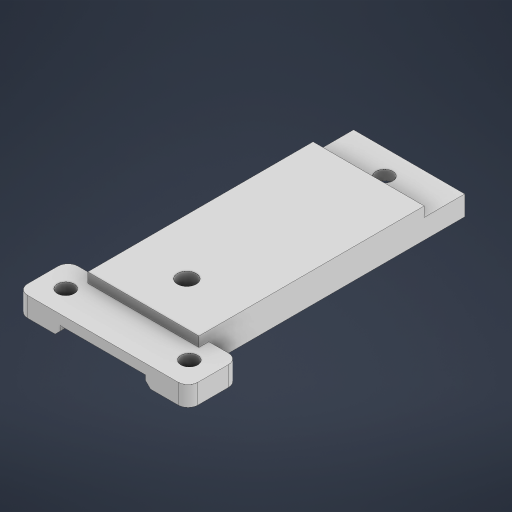
# Autodesk Inventor part: Zwischenplatte
Saved by Autodesk Inventor 2024.2 (Build 282272000, 272)
## iProperties
Created: 2024-01-03
Part Number: Zwischenplatte
Material: Generisch
Document SubType Name: Modeling
Designer: jacob
Density: 1 g/cm^3
Appearance: Vorgabe
Author: jacob
Autodesk Inventor part; units mm, degrees
ref_plane "YZ Plane" through (0, 0, 0) normal (1, 0, 0) x (0, 1, 0)
ref_plane "XZ Plane" through (0, 0, 0) normal (0, 1, 0) x (-1, 0, 0)
ref_plane "XY Plane" through (0, 0, 0) normal (0, 0, 1) x (1, 0, 0)
sketch "Skizze1" plane through (0, 0, 0) normal (0, 1, 0) x (-1, 0, 0)
  line L0 (17.75, 60) -> (-17.75, 60)
  line L1 (-17.75, 60) -> (-17.75, 0)
  line L2 (-17.75, 0) -> (17.75, 0)
  line L3 (17.75, 0) -> (17.75, 60)
  point P0 (0, 0)
  point P1 (0, 0)
  dimension "d0" = 60
  dimension "d1" = 35.5
  constraints: 8 end point, 2 coincident, 2 parallel, 1 horizontal, 1 midpoint, 1 perpendicular
  measures "d0" distance of L2.end L0.start
  measures "d1" distance of L0.start L0.end
extrude "Extrusion1" add sketch "Skizze1" along normal blind 2
sketch "Skizze3" plane through (0, 2, 0) normal (0, 1, 0) x (1, 0, 0)
  line L0 (-17.75, 0) -> (-17.75, -60) projected
  line L1 (17.75, -60) -> (17.75, 0) projected
  line L2 (-17.75, -51.8) -> (17.75, -51.8)
  line L3 (17.75, -51.8) -> (17.75, -6.2)
  line L4 (-17.75, -6.2) -> (-17.75, -51.8)
  line L5 (17.75, 0) -> (-17.75, 0) projected
  line L6 (-17.75, -6.2) -> (17.75, -6.2)
  point P0 (0, 0)
  point P1 (17.75, -51.8)
  point P2 (0, 0)
  dimension "d71" = 51.8
  dimension "d75" = 6.2
  constraints: 8 end point, 2 perpendicular, 2 point on line, 1 horizontal, 1 midpoint, 1 parallel
  measures "d71" distance between parallel lines of L5 L2
  measures "d75" distance from line of point (0, 0) L6
extrude "Extrusion3" add sketch "Skizze3" along normal blind 2 contours L6 L1 L2 L0
sketch "Skizze6" plane through (0, 0, 0) normal (0, -1, 0) x (1, 0, 0)
  line L0 (-17.75, 60) -> (17.75, 60) projected
  line L1 (11.25, 60) -> (-11.25, 60)
  line L2 (-11.25, 60) -> (-11.25, 0)
  line L3 (-11.25, 0) -> (11.25, 0)
  line L4 (11.25, 0) -> (11.25, 60)
  line L5 (8.65, 60) -> (-8.65, 60)
  line L6 (-8.65, 60) -> (-8.65, 0)
  line L7 (-8.65, 0) -> (8.65, 0)
  line L8 (8.65, 0) -> (8.65, 60)
  line L9 (0, -15.6) -> (0, 72.6) projected
  line L10 (17.75, 0) -> (-17.75, 0) projected
  point P0 (0, 0)
  point P1 (0, 60)
  point P2 (0, -1)
  point P3 (0, 60)
  point P4 (0, 0)
  point P5 (8.65, 0)
  point P6 (-8.65, 0)
  dimension "d24" = 17.3
  dimension "d25" = 22.5
  constraints: 16 end point, 4 parallel, 3 horizontal, 3 midpoint, 2 perpendicular, 2 point on line, 2 vertical alignment, 2 other
  measures "d24" distance between parallel lines of L8 L6
  measures "d25" distance between parallel lines of L2 L4
extrude "Extrusion6" add sketch "Skizze6" along normal blind 2 contours L0 L6 L3 L2 | L0 L4 L3 L8
sketch "Skizze7" plane through (0, -2, 0) normal (0, -1, 0) x (1, 0, 0)
  line L0 (17.75, 0) -> (11.25, 0)
  line L1 (11.25, 0) -> (11.25, 60)
  line L2 (11.25, 60) -> (17.75, 60)
  line L3 (17.75, 60) -> (17.75, 0)
  point P0 (0, 0)
  dimension "d31" = 6.5
  constraints: 8 end point, 2 coincident, 2 parallel, 1 horizontal, 1 perpendicular
  measures "d31" distance between parallel lines of L3 L1
extrude "Extrusion7" cut sketch "Skizze7" against normal through all
mirror "Spiegeln2" about plane through (0, 0, 0) normal (1, 0, 0) of "Extrusion7"
sketch "Skizze9" plane through (0, 0, 0) normal (0, -1, 0) x (1, 0, 0)
  line L0 (0, -12) -> (0, 72) projected
  line L1 (-11.25, 51.8) -> (-11.25, 60) projected
  line L2 (11.25, 6.2) -> (11.25, 0) projected
  line L3 (-11.25, 60) -> (11.25, 60) projected
  line L4 (11.25, 51.8) -> (-11.25, 51.8) projected
  line L5 (11.25, 60) -> (11.25, 51.8) projected
  line L6 (-11.25, 0) -> (-11.25, 6.2) projected
  line L7 (-11.25, 6.2) -> (11.25, 6.2) projected
  line L8 (11.25, 0) -> (-11.25, 0) projected
  point P0 (0, 0)
  point P1 (0, 3)
  point P2 (0, 0)
  dimension "d79" = 3
  constraints: 1 midpoint, 1 point on line
  measures "d79" distance of point (0, 3) point (0, 0)
hole "Bohrung1" at (0, 0, 3) direction (0, 1, 0) diameter 3.4 depth 4 clearance for "Flachkopfmaschinenschraube" size "M3" standard "ANSI Metrisches M Profil"
sketch "Skizze10" plane through (0, 4, 0) normal (0, 1, 0) x (1, 0, 0)
  line L0 (0, 12) -> (0, -72) projected
  circle A0 centre (0, -3) radius 1.7 projected
  point P0 (0, 0)
  point P1 (0, -43)
  dimension "d46" = 40
  constraints: 1 point on line
  measures "d46" distance of point (0, -43) A0.centre
hole "Bohrung2" at (0, 4, 43) direction (0, -1, 0) diameter 3.4 depth 4 counterbore diameter 3.8 counterbore depth 3.5
sketch "Skizze11" plane through (-11.25, 4, 9.2) normal (-1, 0, 0) x (0, 0, 1)
  line L0 (50.8, -6) -> (42.6, -6)
  line L1 (42.6, -6) -> (42.6, -2)
  line L2 (42.6, -2) -> (50.8, -2)
  line L3 (50.8, -2) -> (50.8, -6)
  point P0 (-9.2, -4)
  point P1 (42.6, -2)
  constraints: 8 end point, 3 coincident, 2 parallel, 1 horizontal, 1 perpendicular
extrude "Extrusion9" add sketch "Skizze11" along normal blind 6
sketch "Skizze12" plane through (0, -2, 0) normal (0, -1, 0) x (1, 0, 0)
  line L0 (-8.65, 60) -> (-17.25, 60) projected
  line L1 (-11.25, 51.8) -> (-11.25, 0) projected
  line L2 (-11.25, 51.8) -> (-17.25, 51.8) projected
  point P0 (0, 0)
  point P1 (-12.5, 55)
  point P2 (-11.25, 9.2)
  dimension "d80" = 1.25
  dimension "d81" = 3.2
  measures "d80" distance from line of L1 point (-12.5, 55)
  measures "d81" distance from line of L2 point (-12.5, 55)
hole "Bohrung3" at (-12.5, -2, 55) direction (0, 1, 0) diameter 3.4 depth 4 countersink diameter 5 countersink angle 90 clearance for "Flachkopfmaschinenschraube" size "M3" standard "ANSI Metrisches M Profil"
sketch "Skizze13" plane through (-11.25, -2, 51.8) normal (0, 0, -1) x (-1, 0, 0)
  line L0 (0, 0) -> (0, 4) projected
  line L1 (0, 0) -> (6, 0) projected
  line L2 (6, 4) -> (6, 0) projected
  line L3 (0, 4) -> (6, 4) projected
  point P0 (-11.25, 2)
extrude "Extrusion10" add sketch "Skizze13" along normal blind 2
fillet "Rundung1" radius 2 2 edges at (-17.25, 0, 60) (-17.25, 0, 49.8)
mirror "Spiegeln6" about plane through (0, 0, 0) normal (1, 0, 0) of "Extrusion9", "Bohrung3", "Extrusion10", "Rundung1"
chamfer "Fasen3" distance 1 angle 45 2 edges at (-8.65, -2, 30) (8.65, -2, 30)
sketch "Skizze14" plane through (8.65, 0, 0) normal (0, 0, -1) x (-1, 0, 0)
  line L0 (0, -1) -> (-1, -2) projected
  line L1 (0, 0) -> (0, -1) projected
  line L2 (0, 0) -> (17.3, 0) projected
  line L3 (17.3, 0) -> (17.3, -1) projected
  line L4 (18.3, -2) -> (17.3, -1) projected
  line L5 (19.9, -2) -> (18.3, -2) projected
  line L6 (19.9, -2) -> (19.9, 2) projected
  line L7 (-2.6, 2) -> (19.9, 2) projected
  line L8 (-2.6, 2) -> (-2.6, -2) projected
  line L9 (-1, -2) -> (-2.6, -2) projected
  point P0 (8.65, 0)
extrude "Extrusion11" add sketch "Skizze14" along normal blind 2
